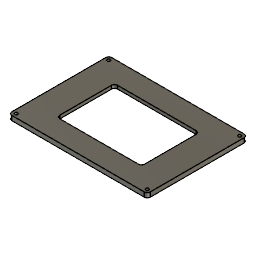
Lid V3.0 (Autodesk Fusion 360 design; units mm, degrees)
part number: 2026-01-29-14-58-12-979
Autodesk Fusion 360 part; units mm, degrees
note: some values were not read from the file. Set by a fixed rule: which sketch regions a step uses.
sketch "Sketch2" plane through (0, 0, 0) normal (0, 0, 1) x (1, 0, 0)
  line L0 (-46, 50) -> (126, 50)
  line L1 (130, 46) -> (130, -76)
  line L2 (126, -80) -> (-46, -80)
  line L3 (-50, -76) -> (-50, 46)
  circle A0 centre (-45, 45) radius 2
  line L4 (40, -80) -> (40, 50) construction
  line L5 (-50, -15) -> (130, -15) construction
  arc A1 (-46, 50) -> (-50, 46) centre (-46, 46) ccw
  circle A2 centre (125, 45) radius 2
  arc A3 (130, 46) -> (126, 50) centre (126, 46) ccw
  circle A4 centre (125, -75) radius 2
  arc A5 (126, -80) -> (130, -76) centre (126, -76) ccw
  circle A6 centre (-45, -75) radius 2
  arc A7 (-50, -76) -> (-46, -80) centre (-46, -76) ccw
  point P0 (-50, 50)
  point P1 (130, 50)
  dimension "d3" = 4
  dimension "d4" = 5
  dimension "d5" = 5
  dimension "d6" = 4
  dimension "d63" = 180
  dimension "d64" = 130
  constraint horizontal L0
  constraint vertical L1
  constraint horizontal L2
  constraint vertical L3
  constraint coincident L0 L4.end
  constraint coincident L3 L5.start
  constraint coincident P0 L0
  constraint coincident P0 L3
  constraint tangent L0 A1
  constraint tangent L3 A1
  constraint symmetric P0 L4 P1
  constraint symmetric A0 L4 A2
  constraint symmetric L4 L0.start L0.end
  constraint symmetric L4 L3.end L1.start
  constraint symmetric L4 A1 A3
  constraint coincident L1 L5.end
  constraint symmetric A0 L5 A6
  constraint symmetric L5 L0.start L2.end
  constraint symmetric L5 L3.end L3.start
  constraint symmetric L5 A1 A7
  constraint symmetric L5 L1.start L1.end
  constraint symmetric L5 L0.end L2.start
  constraint symmetric L5 A2 A4
  constraint symmetric L5 A3 A5
  constraint coincident L2 L4.start
  measures "d3" diameter of A0
  measures "d4" distance of L0 A0.centre
  measures "d5" distance of L3 A0.centre
  measures "d6" radius of A1
  measures "d63" distance of L1 L3
  measures "d64" distance of L0 L2
extrude "Extrude1" add sketch "Sketch2" along normal blind 6
sketch "Sketch3" plane through (0, 0, 0) normal (0, 0, -1) x (1, 0, 0)
  circle A0 centre (125, 75) radius 2
  circle A1 centre (-45, 75) radius 2
  circle A2 centre (-45, -45) radius 2
  circle A3 centre (125, -45) radius 2
  arc A4 (-50, -46) -> (-46, -50) centre (-46, -46) ccw
  line L0 (-46, -50) -> (126, -50)
  arc A5 (126, -50) -> (130, -46) centre (126, -46) ccw
  line L1 (130, -46) -> (130, 76)
  arc A6 (130, 76) -> (126, 80) centre (126, 76) ccw
  line L2 (126, 80) -> (-46, 80)
  arc A7 (-46, 80) -> (-50, 76) centre (-46, 76) ccw
  line L3 (-50, 76) -> (-50, -46)
  line L4 (40, 80) -> (40, -50) construction
  line L5 (130, 15) -> (-50, 15) construction
  line L6 (119.9494, -39.9494) -> (-39.9494, -39.9494) construction
  line L7 (-39.9494, -39.9494) -> (-39.9494, 69.9494) construction
  line L8 (-39.9494, 69.9494) -> (119.9494, 69.9494) construction
  line L9 (119.9494, 69.9494) -> (119.9494, -39.9494) construction
  line L10 (119.9494, -39.9494) -> (-39.9494, 69.9494) construction
  line L11 (-39.9494, -39.9494) -> (119.9494, 69.9494) construction
  line L12 (108.2459, -41.3839) -> (-28.2459, -41.3839)
  line L13 (-41.3839, -28.2459) -> (-41.3839, 58.2459)
  line L14 (-28.2459, 71.3839) -> (108.2459, 71.3839)
  line L15 (121.3839, 58.2459) -> (121.3839, -28.2459)
  line L16 (95.6336, -23.5438) -> (-41.3839, 71.3839) construction
  line L17 (-38.6963, -33.1786) -> (83.6146, 41.7012) construction
  line L18 (-38.5149, -28.2459) -> (-38.5149, 58.2459)
  line L19 (-28.2459, 68.5149) -> (108.2459, 68.5149)
  line L20 (118.5149, 58.2459) -> (118.5149, -28.2459)
  line L21 (104.513, -28.9713) -> (-38.5149, 68.5149) construction
  line L22 (-36.0332, -30.305) -> (80.8211, 39.3236) construction
  arc A8 (-28.2459, 68.5149) -> (-38.5149, 58.2459) centre (-28.2459, 58.2459) ccw
  arc A9 (-28.2459, 71.3839) -> (-41.3839, 58.2459) centre (-28.2459, 58.2459) ccw
  arc A10 (118.5149, 58.2459) -> (108.2459, 68.5149) centre (108.2459, 58.2459) ccw
  arc A11 (121.3839, 58.2459) -> (108.2459, 71.3839) centre (108.2459, 58.2459) ccw
  arc A12 (-38.5149, -28.2459) -> (-28.2459, -38.5149) centre (-28.2459, -28.2459) ccw
  arc A13 (-41.3839, -28.2459) -> (-28.2459, -41.3839) centre (-28.2459, -28.2459) ccw
  arc A14 (108.2459, -38.5149) -> (118.5149, -28.2459) centre (108.2459, -28.2459) ccw
  arc A15 (108.2459, -41.3839) -> (121.3839, -28.2459) centre (108.2459, -28.2459) ccw
  line L23 (108.2459, -38.5149) -> (-28.2459, -38.5149)
  point P0 (40, 15)
  point P1 (40, 15)
  point P2 (40, 15)
  point P3 (40, 15)
  point P4 (40, 15)
  dimension "d25" = 159.8988
  dimension "d27" = 109.8988
  dimension "d28" = 1.4345
  dimension "d29" = 1.4345
  dimension "d30" = 1.4345
  dimension "d31" = 1.4345
  dimension "d44" = 10.269
  dimension "d45" = 13.138
  constraint midpoint L2 L4.start
  constraint midpoint L0 L4.end
  constraint midpoint L1 L5.start
  constraint midpoint L3 L5.end
  constraint midpoint L4 P4
  constraint coincident P4 P3
  constraint horizontal L6
  constraint perpendicular L6 L7
  constraint parallel L6 L8
  constraint parallel L7 L9
  constraint coincident L10 P4
  constraint coincident L11 P4
  constraint horizontal L12
  constraint perpendicular L12 L13
  constraint parallel L12 L14
  constraint parallel L13 L15
  constraint coincident L16 P4
  constraint coincident L17 P4
  constraint perpendicular L18 L23
  constraint parallel L19 L23
  constraint parallel L18 L20
  constraint coincident L21 P4
  constraint coincident L22 P4
  constraint coincident L21.end L19
  constraint coincident L21.end L18
  constraint tangent L19 A8
  constraint tangent L18 A8
  constraint coincident L16.end L14
  constraint coincident L16.end L13
  constraint tangent L14 A9
  constraint tangent L13 A9
  constraint symmetric L4 L19.start L19.end
  constraint symmetric L4 L18.end L20.start
  constraint symmetric L4 A8 A10
  constraint symmetric L4 L14.start L14.end
  constraint symmetric L4 L13.end L15.start
  constraint symmetric L4 A9 A11
  constraint symmetric L5 L19.start A12.end
  constraint symmetric L5 L18.end L18.start
  constraint symmetric L5 A8 A12
  constraint symmetric L5 L14.start L12.end
  constraint symmetric L5 L13.end L13.start
  constraint symmetric L5 A9 A13
  constraint symmetric L5 L19.end A14.start
  constraint symmetric L5 L20.start L20.end
  constraint symmetric L5 A10 A14
  constraint symmetric L5 L14.end L12.start
  constraint symmetric L5 L15.start L15.end
  constraint symmetric L5 A11 A15
  measures "d25" distance of L7.end L8.end
  measures "d27" distance of L6.end L7.end
  measures "d28" distance of L9 L15
  measures "d29" distance of L8 L14
  measures "d30" distance of L8 L19
  measures "d31" distance of L9 L20
  measures "d44" radius of A8
  measures "d45" radius of A9
extrude "Extrude4" add sketch "Sketch3" along normal blind 1.424 contours L12 L13 L14 L15 A9 A11 A13 A15
draft "Draft3" angle 10 neutral plane through (0, 0, -1.424) pull (0, 0, -1) 16 faces at (62.7486, -68.5149, -0.9493) (117.7793, -62.0625, -0.9493) (118.5149, -29.4153, -0.4747) (115.6779, 35.3323, -0.9493) (62.7486, 38.5149, -0.4747) (-32.9514, 37.3734, -0.9493) (-38.5149, -29.4153, -0.9493) (-35.6779, -65.3323, -0.9493) (-41.3839, -0.5847, -0.4747) (-33.1288, 40.4428, -0.9493) (17.2514, 41.3839, -0.9493) (116.3673, 38.5731, -0.9493) (121.3839, -29.4153, -0.9493) (119.6238, -64.8149, -0.9493) (62.7486, -71.3839, -0.9493) (-38.9478, -65.8667, -0.9493)
sketch "Sketch5" plane through (0, 0, -1.424) normal (0, 0, -1) x (1, 0, 0)
  line L0 (-28.2459, 68.5149) -> (108.2459, 68.5149)
  line L1 (118.5149, 58.2459) -> (118.5149, -28.2459)
  line L2 (108.2459, -38.5149) -> (-28.2459, -38.5149)
  line L3 (-38.5149, -28.2459) -> (-38.5149, 58.2459)
  line L4 (108.2459, 71.3839) -> (-28.2459, 71.3839)
  line L5 (-41.3839, 58.2459) -> (-41.3839, -28.2459)
  line L6 (-28.2459, -41.3839) -> (108.2459, -41.3839)
  line L7 (121.3839, -28.2459) -> (121.3839, 58.2459)
  line L8 (40, 71.3839) -> (40, -41.3839) construction
  line L9 (121.3839, 15) -> (-41.3839, 15) construction
  line L10 (119.9494, -39.9494) -> (-39.9494, -39.9494) construction
  line L11 (-39.9494, -39.9494) -> (-39.9494, 69.9494) construction
  line L12 (-39.9494, 69.9494) -> (119.9494, 69.9494) construction
  line L13 (119.9494, 69.9494) -> (119.9494, -39.9494) construction
  line L14 (119.9494, -39.9494) -> (-39.9494, 69.9494) construction
  line L15 (-39.9494, -39.9494) -> (119.9494, 69.9494) construction
  line L16 (108.2459, -40.8839) -> (-28.2459, -40.8839)
  line L17 (-40.8839, -28.2459) -> (-40.8839, 58.2459)
  line L18 (-28.2459, 70.8839) -> (108.2459, 70.8839)
  line L19 (120.8839, 58.2459) -> (120.8839, -28.2459)
  line L20 (98.0985, -25.1411) -> (-40.8839, 70.8839) construction
  line L21 (-40.8839, -40.8839) -> (98.0985, 55.1411) construction
  line L22 (108.2459, -39.0149) -> (-28.2459, -39.0149)
  line L23 (-39.0149, -28.2459) -> (-39.0149, 58.2459)
  line L24 (119.0149, 58.2459) -> (119.0149, -28.2459)
  line L25 (97.1479, -24.0666) -> (-39.0149, 69.0149) construction
  line L26 (-39.0149, -39.0149) -> (97.1479, 54.0666) construction
  arc A0 (118.5149, 58.2459) -> (108.2459, 68.5149) centre (108.2459, 58.2459) ccw
  arc A1 (108.2459, -38.5149) -> (118.5149, -28.2459) centre (108.2459, -28.2459) ccw
  arc A2 (-38.5149, -28.2459) -> (-28.2459, -38.5149) centre (-28.2459, -28.2459) ccw
  arc A3 (-28.2459, 68.5149) -> (-38.5149, 58.2459) centre (-28.2459, 58.2459) ccw
  arc A4 (-41.3839, -28.2459) -> (-28.2459, -41.3839) centre (-28.2459, -28.2459) ccw
  arc A5 (108.2459, -41.3839) -> (121.3839, -28.2459) centre (108.2459, -28.2459) ccw
  arc A6 (121.3839, 58.2459) -> (108.2459, 71.3839) centre (108.2459, 58.2459) ccw
  arc A7 (-28.2459, 71.3839) -> (-41.3839, 58.2459) centre (-28.2459, 58.2459) ccw
  arc A8 (-28.2459, 69.0149) -> (-39.0149, 58.2459) centre (-28.2459, 58.2459) ccw
  arc A9 (-28.2459, 70.8839) -> (-40.8839, 58.2459) centre (-28.2459, 58.2459) ccw
  arc A10 (119.0149, 58.2459) -> (108.2459, 69.0149) centre (108.2459, 58.2459) ccw
  arc A11 (120.8839, 58.2459) -> (108.2459, 70.8839) centre (108.2459, 58.2459) ccw
  line L27 (-28.2459, 69.0149) -> (108.2459, 69.0149)
  arc A12 (108.2459, -39.0149) -> (119.0149, -28.2459) centre (108.2459, -28.2459) ccw
  arc A13 (108.2459, -40.8839) -> (120.8839, -28.2459) centre (108.2459, -28.2459) ccw
  arc A14 (-39.0149, -28.2459) -> (-28.2459, -39.0149) centre (-28.2459, -28.2459) ccw
  arc A15 (-40.8839, -28.2459) -> (-28.2459, -40.8839) centre (-28.2459, -28.2459) ccw
  point P0 (40, 15)
  point P1 (40, 15)
  point P2 (40, 15)
  dimension "d36" = 159.8988
  dimension "d37" = 109.8988
  dimension "d38" = 0.9345
  dimension "d39" = 0.9345
  dimension "d40" = 0.9345
  dimension "d41" = 0.9345
  dimension "d50" = 10.769
  dimension "d51" = 12.638
  constraint midpoint L4 L8.start
  constraint midpoint L6 L8.end
  constraint midpoint L7 L9.start
  constraint midpoint L5 L9.end
  constraint horizontal L10
  constraint perpendicular L10 L11
  constraint parallel L10 L12
  constraint parallel L11 L13
  constraint coincident L14 P2
  constraint coincident L15 P2
  constraint midpoint L8 P2
  constraint horizontal L16
  constraint perpendicular L16 L17
  constraint parallel L16 L18
  constraint parallel L17 L19
  constraint coincident L20 P2
  constraint coincident L21 P2
  constraint coincident P2 P1
  constraint horizontal L22
  constraint perpendicular L22 L23
  constraint parallel L22 L27
  constraint parallel L23 L24
  constraint coincident L25 P2
  constraint coincident L26 P2
  constraint coincident L26.start L23
  constraint coincident L26.start L22
  constraint coincident L21.start L17
  constraint coincident L21.start L16
  constraint coincident L25.end L27
  constraint coincident L25.end L23
  constraint tangent A8 L27
  constraint tangent L23 A8
  constraint coincident L20.end L18
  constraint coincident L20.end L17
  constraint tangent L18 A9
  constraint tangent L17 A9
  constraint symmetric L8 A8.start A10.end
  constraint symmetric L8 L23.end L24.start
  constraint symmetric L8 A8 A10
  constraint symmetric L8 L18.start L18.end
  constraint symmetric L8 L17.end L19.start
  constraint symmetric L8 A9 A11
  constraint symmetric L9 A10.end L22.start
  constraint symmetric L9 L24.start L24.end
  constraint symmetric L9 A10 A12
  constraint symmetric L9 L18.end L16.start
  constraint symmetric L9 L19.start L19.end
  constraint symmetric L9 A11 A13
  constraint symmetric L9 A8.start L22.end
  constraint symmetric L9 L23.end L23.start
  constraint symmetric L9 A8 A14
  constraint symmetric L9 L18.start L16.end
  constraint symmetric L9 L17.end L17.start
  constraint symmetric L9 A9 A15
  constraint coincident L23.start A14.start
  constraint coincident L17.start A15.start
  constraint coincident L22.end A14.end
  constraint coincident L16.end A15.end
  measures "d36" distance of L11.end L12.end
  measures "d37" distance of L10.end L11.end
  measures "d38" distance of L13 L19
  measures "d39" distance of L13 L24
  measures "d40" distance of L10 L16
  measures "d41" distance of L10 L22
  measures "d50" radius of A8
  measures "d51" radius of A9
extrude "Extrude6" cut sketch "Sketch5" against normal blind 1.424 contours L16 L17 L18 L19 A9 A11 A13 A15
extrude "Extrude7" cut 1 faces at (17.2514, 2.7546, 0) along direction (0, 0, 1) blind 0.5
sketch "Sketch6" plane through (0, 0, 0.5) normal (0, 0, -1) x (1, 0, 0)
  line L0 (108.2459, 68.2638) -> (-28.2459, 68.2638)
  arc A0 (-28.2459, 68.2638) -> (-38.2638, 58.2459) centre (-28.2459, 58.2459) ccw
  line L1 (-38.2638, 58.2459) -> (-38.2638, -28.2459)
  arc A1 (-38.2638, -28.2459) -> (-28.2459, -38.2638) centre (-28.2459, -28.2459) ccw
  line L2 (-28.2459, -38.2638) -> (108.2459, -38.2638)
  arc A2 (108.2459, -38.2638) -> (118.2638, -28.2459) centre (108.2459, -28.2459) ccw
  line L3 (118.2638, -28.2459) -> (118.2638, 58.2459)
  arc A3 (118.2638, 58.2459) -> (108.2459, 68.2638) centre (108.2459, 58.2459) ccw
  line L4 (40, 68.2638) -> (40, -38.2638) construction
  line L5 (-38.2638, 15) -> (118.2638, 15) construction
  line L6 (96, -27.5) -> (-16, -27.5)
  line L7 (-20, -23.5) -> (-20, 53.5)
  line L8 (-16, 57.5) -> (96, 57.5)
  line L9 (100, 53.5) -> (100, -23.5)
  line L10 (100, -27.5) -> (-20, 57.5) construction
  line L11 (-20, -27.5) -> (100, 57.5) construction
  arc A4 (-16, 57.5) -> (-20, 53.5) centre (-16, 53.5) ccw
  arc A5 (100, 53.5) -> (96, 57.5) centre (96, 53.5) ccw
  arc A6 (96, -27.5) -> (100, -23.5) centre (96, -23.5) ccw
  arc A7 (-20, -23.5) -> (-16, -27.5) centre (-16, -23.5) ccw
  point P0 (40, 15)
  dimension "d58" = 120
  dimension "d59" = 85
  dimension "d68" = 4
  dimension "d69" = 4
  dimension "d70" = 4
  dimension "d71" = 4
  constraint midpoint L0 L4.start
  constraint midpoint L2 L4.end
  constraint midpoint L1 L5.start
  constraint midpoint L3 L5.end
  constraint horizontal L6
  constraint perpendicular L6 L7
  constraint parallel L6 L8
  constraint parallel L7 L9
  constraint coincident L10 P0
  constraint coincident L11 P0
  constraint midpoint L5 P0
  constraint coincident L10.end L8
  constraint coincident L10.end L7
  constraint tangent L8 A4
  constraint tangent L7 A4
  constraint coincident L11.end L8
  constraint coincident L11.end L9
  constraint tangent L8 A5
  constraint tangent L9 A5
  constraint coincident L10.start L9
  constraint coincident L10.start L6
  constraint tangent L9 A6
  constraint tangent L6 A6
  constraint coincident L11.start L7
  constraint coincident L11.start L6
  constraint tangent L7 A7
  constraint tangent L6 A7
  measures "d58" distance of L10.end L11.end
  measures "d59" distance of L11.start L10.end
  measures "d68" radius of A4
  measures "d69" radius of A5
  measures "d70" radius of A6
  measures "d71" radius of A7
extrude "Extrude8" cut sketch "Sketch6" against normal blind 1.1 contours L6 L7 L8 L9 A4 A5 A6 A7
sketch "Sketch7" plane through (0, 0, 1.6) normal (0, 0, -1) x (1, 0, 0)
  line L0 (96, 57.5) -> (-16, 57.5)
  line L1 (-20, 53.5) -> (-20, -23.5)
  line L2 (-16, -27.5) -> (96, -27.5)
  line L3 (100, -23.5) -> (100, 53.5)
  line L4 (40, 57.5) -> (40, -27.5) construction
  line L5 (100, 15) -> (-20, 15) construction
  line L6 (91, -22.5) -> (-11, -22.5)
  line L7 (-15, -18.5) -> (-15, 48.5)
  line L8 (-11, 52.5) -> (91, 52.5)
  line L9 (95, 48.5) -> (95, -18.5)
  line L10 (95, -22.5) -> (-15, 52.5) construction
  line L11 (-15, -22.5) -> (95, 52.5) construction
  arc A0 (-16, 57.5) -> (-20, 53.5) centre (-16, 53.5) ccw
  arc A1 (-20, -23.5) -> (-16, -27.5) centre (-16, -23.5) ccw
  arc A2 (96, -27.5) -> (100, -23.5) centre (96, -23.5) ccw
  arc A3 (100, 53.5) -> (96, 57.5) centre (96, 53.5) ccw
  arc A4 (-11, 52.5) -> (-15, 48.5) centre (-11, 48.5) ccw
  arc A5 (95, 48.5) -> (91, 52.5) centre (91, 48.5) ccw
  arc A6 (91, -22.5) -> (95, -18.5) centre (91, -18.5) ccw
  arc A7 (-15, -18.5) -> (-11, -22.5) centre (-11, -18.5) ccw
  point P0 (40, 15)
  dimension "d62" = 110
  dimension "d65" = 75
  dimension "d72" = 4
  dimension "d73" = 4
  dimension "d74" = 4
  dimension "d75" = 4
  constraint midpoint L0 L4.start
  constraint midpoint L2 L4.end
  constraint midpoint L3 L5.start
  constraint midpoint L1 L5.end
  constraint horizontal L6
  constraint perpendicular L6 L7
  constraint parallel L6 L8
  constraint parallel L7 L9
  constraint coincident L10 P0
  constraint coincident L11 P0
  constraint midpoint L4 P0
  constraint coincident L10.end L8
  constraint coincident L10.end L7
  constraint tangent L8 A4
  constraint tangent L7 A4
  constraint coincident L11.end L9
  constraint coincident L11.end L8
  constraint tangent L9 A5
  constraint tangent L8 A5
  constraint coincident L10.start L9
  constraint coincident L10.start L6
  constraint tangent L9 A6
  constraint tangent L6 A6
  constraint coincident L11.start L6
  constraint coincident L11.start L7
  constraint tangent L6 A7
  constraint tangent L7 A7
  measures "d62" distance of L10.end L11.end
  measures "d65" distance of L11.start L10.end
  measures "d72" radius of A4
  measures "d73" radius of A5
  measures "d74" radius of A6
  measures "d75" radius of A7
extrude "Extrude9" cut sketch "Sketch7" against normal blind 8.4 contours L6 L7 L8 L9 A4 A5 A6 A7
equation "ORingDiameter = 1.78 mm" comment "Diamter of the O ring"
equation "ORingInnerDiameter = 170 mm" comment "Inner diamter of the o ring bore"
equation "d25 = ( ORingPerimeter - 100 mm ) / 4 + 50 mm"
equation "ORingPerimeter = 2 * 3.1412 * ( ( ORingInnerDiameter / 2 ) + ORingDiameter / 2 )"
equation "d27 = ( ORingPerimeter - 100 mm ) / 4"
equation "d28 = ( ( ORingDiameter * 1.05 ) / 2 ) + 0.5 mm"
equation "d29 = ( ( ORingDiameter * 1.05 ) / 2 ) + 0.5 mm"
equation "d30 = ( ( ORingDiameter * 1.05 ) / 2 ) + 0.5 mm"
equation "d31 = ( ( ORingDiameter * 1.05 ) / 2 ) + 0.5 mm"
equation "d32 = ORingDiameter * 0.8"
equation "d36 = ( ORingPerimeter - 100 mm ) / 4 + 50 mm"
equation "d37 = ( ORingPerimeter - 100 mm ) / 4"
equation "d38 = ( ORingDiameter * 1.05 ) / 2"
equation "d39 = ( ORingDiameter * 1.05 ) / 2"
equation "d40 = ( ORingDiameter * 1.05 ) / 2"
equation "d41 = ( ORingDiameter * 1.05 ) / 2"
equation "d44 = ( ORingDiameter ) * 6 + ORingDiameter * 0.05 - 0.5 mm"
equation "d45 = ( ORingDiameter ) * 6 + ( ORingDiameter * 1.1 ) + 0.5 mm"
equation "d50 = ( ORingDiameter ) * 6 + ORingDiameter * 0.05 - 0.0 mm"
equation "d51 = ( ORingDiameter ) * 6 + ORingDiameter * 1.1 + 0 mm"
equation "d52 = -( ORingDiameter * 0.8 )"
equation "PanelWidth = 85 mm"
equation "PanelLength = 120 mm"
equation "d58 = PanelLength"
equation "d59 = PanelWidth"
equation "d62 = PanelLength - 10 mm"
equation "d65 = PanelWidth - 10 mm"
